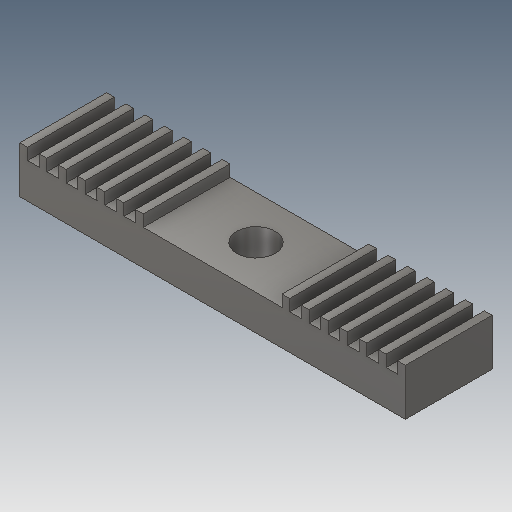
# Autodesk Inventor part: fixador-correia
Saved by Autodesk Inventor 2017 (Build 210142000, 142)
## iProperties
Created: 2018-06-18
Part Number: fixador-correia
Material: Steel, Cast
Document SubType Name: Modeling
Designer: Luiz Gustavo
Density: 7.85 g/cm^3
Appearance: Semi-Polished
Mass: 10.9044 g
Surface Area: 14.2771 cm^2
Volume: 1.38909 cm^3
Author: Luiz Gustavo
Autodesk Inventor part; units mm, degrees
ref_plane "YZ Plane" through (0, 0, 0) normal (1, 0, 0) x (0, 1, 0)
ref_plane "XZ Plane" through (0, 0, 0) normal (0, 1, 0) x (-1, 0, 0)
ref_plane "XY Plane" through (0, 0, 0) normal (0, 0, 1) x (1, 0, 0)
sketch "Sketch1" plane through (0, 0, 0) normal (0, 0, 1) x (1, 0, 0)
  line L0 (-20, 2.425) -> (-19.2, 2.425)
  line L1 (0, -2.425) -> (-20, -2.425)
  line L2 (-20, -2.425) -> (-20, 2.425)
  line L3 (-18, 2.425) -> (-18, 1.225)
  line L4 (-18, 1.225) -> (-19.2, 1.225)
  line L5 (-19.2, 1.225) -> (-19.2, 2.425)
  line L6 (-16, 2.425) -> (-16, 1.225)
  line L7 (-16, 1.225) -> (-17.2, 1.225)
  line L8 (-17.2, 1.225) -> (-17.2, 2.425)
  line L9 (-14, 2.425) -> (-14, 1.225)
  line L10 (-14, 1.225) -> (-15.2, 1.225)
  line L11 (-15.2, 1.225) -> (-15.2, 2.425)
  line L12 (-12, 2.425) -> (-12, 1.225)
  line L13 (-12, 1.225) -> (-13.2, 1.225)
  line L14 (-13.2, 1.225) -> (-13.2, 2.425)
  line L15 (-10, 2.425) -> (-10, 1.225)
  line L16 (-10, 1.225) -> (-11.2, 1.225)
  line L17 (-11.2, 1.225) -> (-11.2, 2.425)
  line L18 (-20, 1.225) -> (0, 1.225) construction
  line L19 (0, 0) -> (-20, 0) construction
  line L20 (-8, 2.425) -> (-8, 1.225)
  line L21 (-8, 1.225) -> (-9.2, 1.225)
  line L22 (-9.2, 1.225) -> (-9.2, 2.425)
  line L23 (0, 1.225) -> (-7.2, 1.225)
  line L24 (-7.2, 1.225) -> (-7.2, 2.425)
  line L25 (-18, 2.425) -> (-17.2, 2.425)
  line L26 (-16, 2.425) -> (-15.2, 2.425)
  line L27 (-14, 2.425) -> (-13.2, 2.425)
  line L28 (-12, 2.425) -> (-11.2, 2.425)
  line L29 (-10, 2.425) -> (-9.2, 2.425)
  line L30 (-8, 2.425) -> (-7.2, 2.425)
  line L31 (0, 1.225) -> (0, -2.425) construction
  line L32 (20, 2.425) -> (19.2, 2.425)
  line L33 (0, -2.425) -> (20, -2.425)
  line L34 (20, -2.425) -> (20, 2.425)
  line L35 (18, 2.425) -> (18, 1.225)
  line L36 (18, 1.225) -> (19.2, 1.225)
  line L37 (19.2, 1.225) -> (19.2, 2.425)
  line L38 (16, 2.425) -> (16, 1.225)
  line L39 (16, 1.225) -> (17.2, 1.225)
  line L40 (17.2, 1.225) -> (17.2, 2.425)
  line L41 (14, 2.425) -> (14, 1.225)
  line L42 (14, 1.225) -> (15.2, 1.225)
  line L43 (15.2, 1.225) -> (15.2, 2.425)
  line L44 (12, 2.425) -> (12, 1.225)
  line L45 (12, 1.225) -> (13.2, 1.225)
  line L46 (13.2, 1.225) -> (13.2, 2.425)
  line L47 (10, 2.425) -> (10, 1.225)
  line L48 (10, 1.225) -> (11.2, 1.225)
  line L49 (11.2, 1.225) -> (11.2, 2.425)
  line L50 (20, 1.225) -> (0, 1.225) construction
  line L51 (0, 0) -> (20, 0) construction
  line L52 (8, 2.425) -> (8, 1.225)
  line L53 (8, 1.225) -> (9.2, 1.225)
  line L54 (9.2, 1.225) -> (9.2, 2.425)
  line L55 (0, 1.225) -> (7.2, 1.225)
  line L56 (7.2, 1.225) -> (7.2, 2.425)
  line L57 (18, 2.425) -> (17.2, 2.425)
  line L58 (16, 2.425) -> (15.2, 2.425)
  line L59 (14, 2.425) -> (13.2, 2.425)
  line L60 (12, 2.425) -> (11.2, 2.425)
  line L61 (10, 2.425) -> (9.2, 2.425)
  line L62 (8, 2.425) -> (7.2, 2.425)
  dimension "d0" = 4.85
  dimension "d3" = 1.2
  dimension "d4" = 0.8
  dimension "d5" = 1.2
  dimension "d6" = 0.8
  dimension "d7" = 1.2
  dimension "d8" = 0.8
  dimension "d9" = 1.2
  dimension "d10" = 0.8
  dimension "d13" = 0.8
  dimension "d14" = 1.2
  dimension "d15" = 0.8
  dimension "d16" = 1.2
  dimension "d17" = 0.8
  dimension "d18" = 40
  dimension "d19" = 3.65
  constraints: 126 end point, 30 symmetric about line, 13 point on line, 11 collinear, 7 horizontal, 7 parallel, 3 midpoint, 2 coincident, 1 vertical
  measures "d0" distance between parallel lines of L1 L0
  measures "d3" distance of L3.end L4.end
  measures "d4" distance between parallel lines of L8 L3
  measures "d5" distance of L6.end L7.end
  measures "d6" distance between parallel lines of L2 L5
  measures "d7" distance of L9.end L10.end
  measures "d8" distance between parallel lines of L6 L11
  measures "d9" distance of L12.end L13.end
  measures "d10" distance between parallel lines of L9 L14
  measures "d13" distance between parallel lines of L12 L17
  measures "d14" distance between parallel lines of L17 L15
  measures "d15" distance between parallel lines of L15 L22
  measures "d16" distance between parallel lines of L22 L20
  measures "d17" distance between parallel lines of L20 L24
  measures "d18" diameter of L2 L31
  measures "d19" distance between parallel lines of L1 L18
extrude "Extrusion1" add sketch "Sketch1" along normal mid plane 9
sketch "Sketch2" plane through (0, 0, 0) normal (0, 1, 0) x (-1, 0, 0)
  circle A0 centre (0, 0) radius 2.2937
  circle A1 centre (0, 0) radius 2
  dimension "d22" = 4
  constraints: 2 centre point, 2 coincident
  measures "d22" diameter of A1
extrude "Extrusion2" cut sketch "Sketch2" along normal through all both and the other way through all contours A1
equation "\"d5\" = d3"
equation "\"d7\" = d3"
equation "\"d8\" = d4"
equation "\"d9\" = d3"
equation "\"d10\" = d4"
equation "\"d13\" = d4"
equation "\"d14\" = d3"
equation "\"d15\" = d4"
equation "\"d16\" = d3"
equation "\"d17\" = d4"
body "Solid1"
